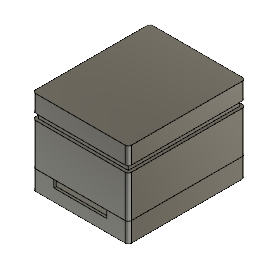
Weave pedal second pass v10 (Autodesk Fusion 360 design; units mm, degrees)
Autodesk Fusion 360 part; units mm, degrees
note: some values were not read from the file. Chosen so that the rebuilt part matches the saved one: which bodies a step acts on; which face or edge a step refers to.
sketch "Sketch1" plane through (0, 0, 0) normal (0, 0, 1) x (1, 0, 0)
  line L0 (39, 47.75) -> (-39, 47.75)
  line L1 (-39, 47.75) -> (-39, -47.75)
  line L2 (-39, -47.75) -> (39, -47.75)
  line L3 (39, -47.75) -> (39, 47.75)
  line L4 (39, 47.75) -> (-39, -47.75) construction
  line L5 (-39, 47.75) -> (39, -47.75) construction
  dimension "d1" = 78
  dimension "d2" = 95.5
  constraint horizontal L0
  constraint perpendicular L0 L1
  constraint parallel L0 L2
  constraint parallel L1 L3
  constraint coincident L4 origin
  constraint coincident L5 origin
  measures "d1" distance of L1.end L2.end
  measures "d2" distance of L0.end L1.end
sketch "Sketch3" plane through (0, 0, 0) normal (1, 0, 0) x (0, 1, 0)
  line L0 (-55, 16) -> (55, 16)
  dimension "d73" = 16
  constraint horizontal L0
  measures "d73" distance of origin L0
extrude "Extrude1" add sketch "Sketch1" along normal blind 50 makes body 1
fillet "Fillet1" radius 2.5 4 edges at (39, -47.75, 25) (-39, -47.75, 25) (39, 47.75, 25) (-39, 47.75, 25) on bodies 1
split "Split1" by curves path "Sketch3" along L0 bodies 1 makes body 2 at (-13, 15.0833, 0)
sketch "Sketch4" plane through (0, 0, 50) normal (0, 0, 1) x (-1, 0, 0)
  arc A0 (36.5, -47.75) -> (39, -45.25) centre (36.5, -45.25) ccw
  line L0 (39, -45.25) -> (39, 45.25)
  arc A1 (39, 45.25) -> (36.5, 47.75) centre (36.5, 45.25) ccw
  line L1 (36.5, 47.75) -> (-36.5, 47.75)
  arc A2 (-36.5, 47.75) -> (-39, 45.25) centre (-36.5, 45.25) ccw
  line L2 (-39, 45.25) -> (-39, -45.25)
  arc A3 (-39, -45.25) -> (-36.5, -47.75) centre (-36.5, -45.25) ccw
  line L3 (-36.5, -47.75) -> (36.5, -47.75)
  line L4 (36.5, -45.25) -> (36.5, 45.25)
  line L5 (36.5, 45.25) -> (-36.5, 45.25)
  line L6 (-36.5, 45.25) -> (-36.5, -45.25)
  line L7 (-36.5, -45.25) -> (36.5, -45.25)
  line L8 (34, -42.75) -> (34, 42.75)
  line L9 (34, 42.75) -> (-34, 42.75)
  line L10 (-34, 42.75) -> (-34, -42.75)
  line L11 (-34, -42.75) -> (34, -42.75)
  dimension "d7" = -2.5
  dimension "d8" = -5
extrude "Extrude2" add sketch "Sketch4" along normal blind 10 separate body contours L4 L5 L6 L7 makes body 3
sketch "Sketch5" plane through (0, 0, 50) normal (0, 0, 1) x (-1, 0, 0)
  circle A0 centre (0, 0) radius 6.25
  arc A1 (36.5, -47.75) -> (39, -45.25) centre (36.5, -45.25) ccw
  line L0 (39, -45.25) -> (39, 45.25)
  arc A2 (39, 45.25) -> (36.5, 47.75) centre (36.5, 45.25) ccw
  line L1 (36.5, 47.75) -> (-36.5, 47.75)
  arc A3 (-36.5, 47.75) -> (-39, 45.25) centre (-36.5, 45.25) ccw
  line L2 (-39, 45.25) -> (-39, -45.25)
  arc A4 (-39, -45.25) -> (-36.5, -47.75) centre (-36.5, -45.25) ccw
  line L3 (-36.5, -47.75) -> (36.5, -47.75)
  dimension "d11" = 12.5
  constraint coincident A0.centre origin
  measures "d11" diameter of A0
shell "Shell1" thickness 2 removed faces 1 at (13, -15.0833, 16) on bodies 1
shell "Shell2" thickness 2 removed faces 1 at (13, -15.0833, 16) on bodies 2
extrude "Extrude3" cut sketch "Sketch5" against normal blind 5 contours A0 bodies 1
sketch "Sketch9" plane through (0, -47.75, 0) normal (0, -1, 0) x (1, 0, 0)
  line L0 (36.5, 16) -> (-36.5, 16)
  line L1 (-36.5, 16) -> (-36.5, 0)
  line L2 (-36.5, 0) -> (36.5, 0)
  line L3 (36.5, 0) -> (36.5, 16)
  line L4 (21.5, 16) -> (-21.5, 16)
  line L5 (-21.5, 16) -> (-21.5, 10)
  line L6 (-21.5, 10) -> (21.5, 10)
  line L7 (21.5, 10) -> (21.5, 16)
  line L8 (21.5, 16) -> (-21.5, 10) construction
  line L9 (-21.5, 16) -> (21.5, 10) construction
  point P0 (0, 13)
  dimension "d30" = 43
  dimension "d31" = 6
  dimension "d34" = 15
  dimension "d56" = 10
  constraint horizontal L4
  constraint perpendicular L4 L5
  constraint parallel L4 L6
  constraint parallel L5 L7
  constraint coincident L8 P0
  constraint coincident L9 P0
  measures "d30" distance of L5.end L6.end
  measures "d31" distance of L4.end L5.end
  measures "d34" distance of L3 L7
  measures "d56" distance of L2 L6
sketch "Sketch10" plane through (0, 47.75, 0) normal (0, 1, 0) x (-1, 0, 0)
  line L0 (36.5, 16) -> (-36.5, 16)
  line L1 (-36.5, 16) -> (-36.5, 0)
  line L2 (-36.5, 0) -> (36.5, 0)
  line L3 (36.5, 0) -> (36.5, 16)
  line L4 (21.5, 2) -> (-21.5, 2)
  line L5 (-21.5, 2) -> (-21.5, 6.5)
  line L6 (-21.5, 6.5) -> (21.5, 6.5)
  line L7 (21.5, 6.5) -> (21.5, 2)
  line L8 (21.5, 2) -> (-21.5, 6.5) construction
  line L9 (-21.5, 2) -> (21.5, 6.5) construction
  point P0 (0, 4.25)
  dimension "d37" = 43
  dimension "d38" = 4.5
  dimension "d40" = 2
  dimension "d41" = 15
  constraint horizontal L4
  constraint perpendicular L4 L5
  constraint parallel L4 L6
  constraint parallel L5 L7
  constraint coincident L8 P0
  constraint coincident L9 P0
  measures "d37" distance of L5.end L6.end
  measures "d38" distance of L4.end L5.end
  measures "d40" distance of L2 L4
  measures "d41" distance of L3 L7
ref_plane "WorkPlane1" through (0, 0, 55) normal (0, 0, 1) x (1, 0, 0)
sketch "Sketch11" plane through (0, 0, 55) normal (0, 0, 1) x (1, 0, 0)
  line L0 (39, -47.75) -> (-39, -47.75)
  line L1 (-39, -47.75) -> (-39, 47.75)
  line L2 (-39, 47.75) -> (39, 47.75)
  line L3 (39, 47.75) -> (39, -47.75)
  line L4 (39, -47.75) -> (-39, 47.75) construction
  line L5 (-39, -47.75) -> (39, 47.75) construction
  dimension "d45" = 78
  dimension "d46" = 95.5
  constraint horizontal L0
  constraint perpendicular L0 L1
  constraint parallel L0 L2
  constraint parallel L1 L3
  constraint coincident L4 origin
  constraint coincident L5 origin
  measures "d45" distance of L1.end L2.end
  measures "d46" distance of L0.end L1.end
extrude "Extrude7" add sketch "Sketch11" along normal blind 14 separate body makes body 4
fillet "Fillet2" radius 2.5 4 edges at (39, -47.75, 62) (-39, -47.75, 62) (39, 47.75, 62) (-39, 47.75, 62) on bodies 4
shell "Shell3" thickness 1.7 removed faces 1 at (-13, 15.0833, 55) on bodies 4
sketch "Sketch12" plane through (0, 0, 67.3) normal (0, 0, -1) x (1, 0, 0)
  arc A0 (-37.3, -45.25) -> (-36.5, -46.05) centre (-36.5, -45.25) ccw
  line L0 (-36.5, -46.05) -> (36.5, -46.05)
  arc A1 (36.5, -46.05) -> (37.3, -45.25) centre (36.5, -45.25) ccw
  line L1 (37.3, -45.25) -> (37.3, 45.25)
  arc A2 (37.3, 45.25) -> (36.5, 46.05) centre (36.5, 45.25) ccw
  line L2 (36.5, 46.05) -> (-36.5, 46.05)
  arc A3 (-36.5, 46.05) -> (-37.3, 45.25) centre (-36.5, 45.25) ccw
  line L3 (-37.3, 45.25) -> (-37.3, -45.25)
  circle A4 centre (0, 0) radius 6
  circle A5 centre (0, 0) radius 8
  dimension "d52" = 12
  dimension "d53" = 2
  constraint coincident A4.centre A5.centre
  measures "d52" diameter of A4
extrude "Extrude8" add sketch "Sketch12" along normal blind 10 contours A5 bodies 4
sketch "Sketch13" plane through (0, 0, 2) normal (0, 0, 1) x (-1, 0, 0)
  arc A0 (36.5, -45.75) -> (37, -45.25) centre (36.5, -45.25) ccw
  line L0 (37, -45.25) -> (37, 45.25)
  arc A1 (37, 45.25) -> (36.5, 45.75) centre (36.5, 45.25) ccw
  line L1 (36.5, 45.75) -> (-36.5, 45.75)
  arc A2 (-36.5, 45.75) -> (-37, 45.25) centre (-36.5, 45.25) ccw
  line L2 (-37, 45.25) -> (-37, -45.25)
  arc A3 (-37, -45.25) -> (-36.5, -45.75) centre (-36.5, -45.25) ccw
  line L3 (-36.5, -45.75) -> (36.5, -45.75)
  circle A4 centre (32.075, -42.225) radius 1.325
  circle A5 centre (-33.575, -43.425) radius 1.325
  circle A6 centre (33.875, 41.425) radius 1.325
  circle A7 centre (-33.275, 41.425) radius 1.325
  dimension "d57" = 2.65
  dimension "d58" = 3.525
  dimension "d59" = 4.925
  dimension "d60" = 2.65
  dimension "d61" = 3.425
  dimension "d62" = 2.325
  dimension "d65" = 3.125
  dimension "d66" = 4.325
  dimension "d67" = 2.65
  dimension "d68" = 4.325
  dimension "d69" = 3.725
  dimension "d70" = 2.65
  measures "d57" diameter of A4
  measures "d58" distance of L3 A4.centre
  measures "d59" distance of L0 A4.centre
  measures "d60" diameter of A5
  measures "d61" distance of L2 A5.centre
  measures "d62" distance of L3 A5.centre
  measures "d65" distance of L0 A6.centre
  measures "d66" distance of L1 A6.centre
  measures "d67" diameter of A6
  measures "d68" distance of L1 A7.centre
  measures "d69" distance of L2 A7.centre
  measures "d70" diameter of A7
extrude "Extrude9" add sketch "Sketch13" along normal blind 18 contours A4 | A5 | A6 | A7 bodies 2
extrude "Extrude10" cut sketch "Sketch9" against normal blind 120 contours L0 L4 L5 L6 L7 bodies 2
sketch "Sketch14" plane through (0, 0, 0) normal (0, 0, 1) x (1, 0, 0)
  line L0 (-50, 10) -> (-47, 10)
  line L1 (-47, 10) -> (-47, 2)
  line L2 (-47, 2) -> (-50, 2)
  line L3 (-50, 2) -> (-50, 10)
  dimension "d76" = 3
  dimension "d77" = 8
  constraint horizontal L0
  constraint vertical L1
  constraint horizontal L2
  constraint vertical L3
  measures "d76" distance of L0.start L0.end
  measures "d77" distance of L0.start L2.end
extrude "Extrude11" add sketch "Sketch14" along normal blind 5 separate body makes body 5
copy_body "CopyPasteBodies1" bodies 5 makes body 6
move_body "Move1" bodies 6 to x (1, 0, 0) y (0, 1, 0) z (0, 0, 1) at (-7, 0, 0)
copy_body "CopyPasteBodies2" bodies 5 6 makes body 7 makes body 8
move_body "Move2" bodies 7 8 to x (1, 0, 0) y (0, 1, 0) z (0, 0, 1) at (0, 10, 0)
named bodies: "Top piece", "bottom piece", "Pedal", "Lip", "Tab", "Tab (1)", "Tab (1) (1)", "Tab (1) (1) (1)"
